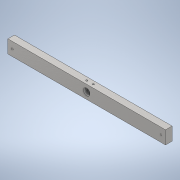
# Autodesk Inventor part: Steering Axle
Saved by Autodesk Inventor 2022 (Build 260153000, 153)
## iProperties
Created: 2021-12-06
Part Number: Steering Axle
Material: Generic
Document SubType Name: Modeling
Designer: Vedic
Density: 1 g/cm^3
Appearance: Default
Author: Vedic
Autodesk Inventor part; units mm, degrees
ref_plane "YZ Plane" through (0, 0, 0) normal (1, 0, 0) x (0, 1, 0)
ref_plane "XZ Plane" through (0, 0, 0) normal (0, 1, 0) x (-1, 0, 0)
ref_plane "XY Plane" through (0, 0, 0) normal (0, 0, 1) x (1, 0, 0)
sketch "Sketch1" plane through (0, 0, 0) normal (0, 0, 1) x (1, 0, 0)
  line L0 (-465.6684, -57.942) -> (143.9316, -57.942)
  line L1 (143.9316, -57.942) -> (143.9316, -108.742)
  line L2 (143.9316, -108.742) -> (-465.6684, -108.742)
  line L3 (-465.6684, -108.742) -> (-465.6684, -57.942)
  line L4 (-465.6684, -83.342) -> (143.9316, -83.342) construction
  circle A0 centre (-448.6631, -83.342) radius 3.175
  circle A1 centre (126.9263, -83.342) radius 3.175
  line L5 (-160.8684, -57.942) -> (-160.8684, -108.742) construction
  point P0 (0, 0)
  dimension "d0" = 575.5894
  dimension "d1" = 287.7947
  dimension "d2" = 609.6
  dimension "d3" = 6.35
  dimension "d4" = 50.8
  constraints: 12 end point, 4 midpoint, 2 centre point, 2 parallel, 2 point on line, 1 equal radius, 1 horizontal, 1 perpendicular
  measures "d0" distance of A1.centre A0.centre
  measures "d1" distance from line of A0.centre L5
  measures "d2" distance of L1.end L2.end
  measures "d3" diameter of A0
  measures "d4" distance of L0.end L1.end
extrude "Extrusion1" add sketch "Sketch1" along normal blind 25.4
sketch "Sketch2" plane through (-465.6684, -57.942, 0) normal (0, 1, 0) x (1, 0, 0)
  line L0 (0, 0) -> (0, -25.4) construction
  line L1 (0, -12.7) -> (609.6, -12.7) construction
  line L2 (609.6, 0) -> (609.6, -25.4) construction
  line L3 (0, -25.4) -> (609.6, -25.4) construction
  line L4 (304.8, -25.4) -> (304.8, 0) construction
  line L5 (0, 0) -> (609.6, 0) construction
  circle A0 centre (292.1, -12.7) radius 3.175
  circle A1 centre (317.5, -12.7) radius 3.175
  point P0 (465.6684, 0)
  dimension "d7" = 6.35
  dimension "d8" = 12.7
  dimension "d9" = 12.7
  constraints: 4 end point, 4 midpoint, 2 centre point, 2 point on line, 1 equal radius
  measures "d7" diameter of A0
  measures "d8" distance from line of L4 A0.centre
  measures "d9" distance from line of L4 A1.centre
extrude "Extrusion2" cut sketch "Sketch2" against normal through all
sketch "Sketch3" plane through (0, 0, 25.4) normal (0, 0, 1) x (1, 0, 0)
  line L0 (-465.6684, -57.942) -> (-465.6684, -108.742) construction
  line L1 (-465.6684, -83.342) -> (143.9316, -83.342) construction
  line L2 (143.9316, -108.742) -> (143.9316, -57.942) construction
  line L3 (143.9316, -57.942) -> (-465.6684, -57.942) construction
  line L4 (-160.8684, -57.942) -> (-160.8684, -108.742) construction
  line L5 (-465.6684, -108.742) -> (143.9316, -108.742) construction
  circle A0 centre (-160.8684, -83.342) radius 12.7
  point P0 (0, 0)
  dimension "d12" = 25.4
  constraints: 5 midpoint, 4 end point, 1 centre point
  measures "d12" diameter of A0
extrude "Extrusion3" cut sketch "Sketch3" against normal through all
equation "\"d1\" = 0.5 * d0"
equation "\"d9\" = d8"
body "Solid1"
